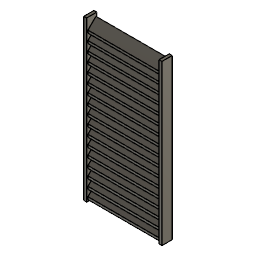
vent (Autodesk Fusion 360 design; units mm, degrees)
part number: 2026-07-17-14-19-08-433
Autodesk Fusion 360 part; units mm, degrees
sketch "Sketch1" plane through (0, 0, 0) normal (1, 0, 0) x (0, 1, 0)
  line L0 (0, 0) -> (9.85, 0)
  line L1 (9.85, 0) -> (9.85, 154.5)
  line L2 (9.85, 154.5) -> (0, 154.5)
  line L3 (0, 154.5) -> (0, 0)
  line L4 (1.2254, 1.5) -> (9.0035, 9.2782)
  line L5 (9.0035, 9.2782) -> (9.0035, 11.7782)
  line L6 (1.2254, 1.5) -> (1.2254, 4)
  line L7 (1.2254, 4) -> (9.0035, 11.7782)
  dimension "d2" = 154.5
  dimension "d4" = 11
  dimension "d6" = 9.85
  dimension "d9" = 1.5
  dimension "d22" = 45
  dimension "d23" = 2.5
  dimension "d24" = 2.5
  dimension "d25" = 1.2254
  constraint vertical L1
  constraint horizontal L2
  constraint vertical L3
  constraint coincident L0.start L3.end
  constraint vertical L5
  constraint parallel L3 L6
  constraint perpendicular L0 L3
  measures "d2" distance of L0.start L2.end
  measures "d4" distance of L4.start L4.end
  measures "d6" distance of L0.start L0.end
  measures "d9" distance of L0 L4.start
  measures "d22" angle of L0 L4
  measures "d23" distance of L4.end L5.end
  measures "d24" distance of L4.start L6.end
  measures "d25" distance of L3 L6
extrude "Extrude1" add sketch "Sketch1" along normal blind 70 contours L4 L5 L6 L7
extrude "Extrude2" add sketch "Sketch1" against normal blind 2.85 contours L0 L1 L2 L3 | L4 L5 L6 L7
pattern_path "PathPattern1" count 17 spacing 8.7289 from (-2.85, 9.85, 5.034) along 1 edges at (-2.85, 9.85, 77.25) of "Extrude1"
sketch "Sketch2" plane through (70, 0, 0) normal (1, 0, 0) x (0, 1, 0)
  line L0 (1.2254, 136.7755) -> (9.0035, 144.5537)
  line L1 (0, 0) -> (10, 0)
  line L2 (10, 0) -> (10, 154.5)
  line L3 (10, 154.5) -> (0, 154.5)
  line L4 (0, 154.5) -> (0, 0)
  dimension "d16" = 10
  dimension "d17" = 154.5
  constraint horizontal L1
  constraint vertical L2
  constraint horizontal L3
  constraint vertical L4
  constraint coincident L1.start L4.end
  measures "d16" distance of L1.start L1.end
  measures "d17" distance of L1.start L3.end
extrude "Extrude4" add sketch "Sketch2" along normal blind 2.85
